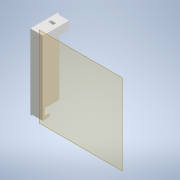
# Autodesk Inventor part: Main
Saved by Autodesk Inventor 2021 (Build 250183000, 183)
## iProperties
Created: 2020-10-20
Part Number: Main
Material: Generic
Document SubType Name: Modeling
Designer: VM
Density: 1 g/cm^3
Appearance: Default
Author: VM
Autodesk Inventor part; units mm, degrees
ref_plane "YZ Plane" through (0, 0, 0) normal (1, 0, 0) x (0, 1, 0)
ref_plane "XZ Plane" through (0, 0, 0) normal (0, 1, 0) x (-1, 0, 0)
ref_plane "XY Plane" through (0, 0, 0) normal (0, 0, 1) x (1, 0, 0)
ref_plane "Work Plane1" through (0, 0, 0) normal (0, 0, 1) x (1, 0, 0)
sketch "Sketch1" plane through (0, 0, 0) normal (0, 0, 1) x (1, 0, 0)
  line L0 (-83, -0.5) -> (-83, -81) projected
  line L1 (2, -82) -> (-93, -82) projected
  line L2 (-95, -2) -> (-95, -80) projected
  line L3 (-83, -81) -> (-96.6, -81)
  line L4 (-96.6, -81) -> (-96.6, 0)
  line L5 (-96.6, 0) -> (-83, 0)
  line L6 (-83, 0) -> (-83, -81)
  point P0 (0, 0)
  dimension "d0" = 1.6
  constraints: 8 end point, 2 parallel, 1 horizontal, 1 perpendicular
  measures "d0" distance between parallel lines of L4 L2
extrude "Extrusion1" add sketch "Sketch1" against normal blind 2.4
sketch "Sketch2" plane through (0, 0, -2.4) normal (0, 0, -1) x (-1, 0, 0)
  line L0 (94, -9.5) -> (83, -9.5) projected
  line L1 (94, -57.961) -> (76.85, -57.961) projected
  line L2 (83, -81) -> (96.6, -81) projected
  line L3 (83, 0) -> (83, -81) projected
  line L4 (96.6, 0) -> (83, 0)
  line L5 (83, 0) -> (83, -9.1)
  line L6 (83, -9.1) -> (96.6, -9.1)
  line L7 (96.6, -9.1) -> (96.6, 0)
  point P0 (0, 0)
  dimension "d3" = 0.4
  constraints: 8 end point, 2 parallel, 1 horizontal, 1 perpendicular, 1 point on line
  measures "d3" distance between parallel lines of L6 L0
extrude "Extrusion2" add sketch "Sketch2" along normal blind 26.2
sketch "Sketch3" plane through (0, 0, -2.4) normal (0, 0, -1) x (-1, 0, 0)
  line L0 (96.6, -81) -> (96.6, -9.1) projected
  line L1 (83, -81) -> (96.6, -81)
  line L2 (96.6, -81) -> (96.6, -77)
  line L3 (96.6, -77) -> (83, -77)
  line L4 (83, -77) -> (83, -81)
  point P0 (0, 0)
  dimension "d6" = 4
  constraints: 8 end point, 2 parallel, 1 horizontal, 1 perpendicular, 1 point on line
  measures "d6" distance between parallel lines of L1 L3
extrude "Extrusion3" add sketch "Sketch3" along normal blind 5
sketch "Sketch4" plane through (-96.6, -81, 0) normal (-1, 0, 0) x (0, 0, 1)
  line L0 (-2.4, 71.9) -> (-2.4, 4) projected
  line L1 (-2.4, 71.9) -> (-10.4, 71.9)
  line L2 (-10.4, 71.9) -> (-10.4, 4)
  line L3 (-10.4, 4) -> (-2.4, 4)
  line L4 (-2.4, 4) -> (-2.4, 71.9)
  line L5 (-2.4, 4) -> (-7.4, 4) projected
  line L6 (-30, 1) -> (-30, 79) projected
  line L7 (-30, 71.9) -> (-13.7225, 71.9)
  line L8 (-13.7225, 71.9) -> (-13.7225, 4)
  line L9 (-13.7225, 4) -> (-30, 4)
  line L10 (-30, 4) -> (-30, 71.9)
  line L11 (-13.7225, 24.3406) -> (-13.7225, 32.8941) projected
  line L12 (-28.6, 71.9) -> (-30, 71.9)
  line L13 (-30, 71.9) -> (-30, 81)
  line L14 (-30, 81) -> (-28.6, 81)
  line L15 (-28.6, 81) -> (-28.6, 71.9)
  point P0 (0, 81)
  dimension "d9" = 8
  constraints: 24 end point, 6 parallel, 3 collinear, 3 horizontal, 3 perpendicular, 1 point on line
  measures "d9" distance of L3.end L2.end
extrude "Extrusion4" add sketch "Sketch4" against normal blind 1.6
sketch "Sketch5" plane through (-96.6, -81, 0) normal (-1, 0, 0) x (0, 0, 1)
  line L0 (-19.219, 23) -> (-0.5, 23) projected
  line L1 (-2, -1) -> (-28, -1) projected
  line L2 (-30, 81) -> (-30, 4) projected
  line L3 (0, 81) -> (0, 0) projected
  line L4 (0, 23) -> (-30, 23)
  line L5 (-30, 23) -> (-30, -1)
  line L6 (-30, -1) -> (0, -1)
  line L7 (0, -1) -> (0, 23)
  point P0 (-0.5, 23)
  point P1 (-28, -1)
  constraints: 8 end point, 2 parallel, 2 point on line, 1 horizontal, 1 perpendicular
extrude "Extrusion5" add sketch "Sketch5" against normal blind 1.6
sketch "Sketch6" plane through (-83, -81, -7.4) normal (0, -1, 0) x (1, 0, 0)
  circle A0 centre (-5.5, 3.4) radius 1.75 projected
  circle A1 centre (-5.5, 3.4) radius 1.5
  point P0 (83, 7.4)
  dimension "d14" = 3
  constraints: 1 centre point, 1 coincident
  measures "d14" diameter of A1
extrude "Extrusion6" add sketch "Sketch6" along normal blind 1.6 contours A1
sketch "Sketch7" plane through (0, 0, -28.6) normal (0, 0, -1) x (-1, 0, 0)
  circle A0 centre (90.5, -5.5) radius 1.75 projected
  circle A1 centre (90.5, -5.5) radius 2
  point P0 (0, 0)
  dimension "d17" = 4
  constraints: 1 centre point, 1 coincident
  measures "d17" diameter of A1
extrude "Extrusion7" cut sketch "Sketch7" against normal blind 12 contours A0 | A1
sketch "Sketch9" plane through (-96.6, 0, 0) normal (0, 1, 0) x (1, 0, 0)
  line L0 (3.1, 16) -> (9.1, 16)
  line L1 (9.1, 16) -> (9.1, 19)
  line L2 (9.1, 19) -> (3.1, 19)
  line L3 (3.1, 19) -> (3.1, 16)
  line L4 (0, 30) -> (1.6, 30) projected
  line L5 (4.1, 28.6) -> (4.1, 16.6) projected
  line L6 (8.1, 28.6) -> (8.1, 16.6) projected
  line L7 (6.1, 36) -> (6.1, -6) projected
  point P0 (96.6, 0)
  dimension "d23" = 3
  dimension "d24" = 6
  dimension "d25" = 11
  dimension "d26" = 3
  constraints: 8 end point, 2 parallel, 1 horizontal, 1 perpendicular
  measures "d23" distance of L2.end L0.start
  measures "d24" distance of L0.start L0.end
  measures "d25" distance between parallel lines of L4 L2
  measures "d26" distance between parallel lines of L7 L3
extrude "Extrusion8" cut sketch "Sketch9" against normal through all
body "Solid1"
